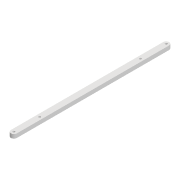
# Autodesk Inventor part: Part_5
Saved by Autodesk Inventor 2022 (Build 260153000, 153)
## iProperties
Created: 2022-04-22
Part Number: Part_5
Material: Generic
Document SubType Name: Modeling
Designer: dell
Density: 1 g/cm^3
Appearance: Default
Mass: 3.67778 g
Surface Area: 33.0626 cm^2
Volume: 3.67778 cm^3
Author: dell
Autodesk Inventor part; units mm, degrees
ref_plane "YZ Plane" through (0, 0, 0) normal (1, 0, 0) x (0, 1, 0)
ref_plane "XZ Plane" through (0, 0, 0) normal (0, 1, 0) x (-1, 0, 0)
ref_plane "XY Plane" through (0, 0, 0) normal (0, 0, 1) x (1, 0, 0)
sketch "Sketch1" plane through (0, 0, 0) normal (0, 1, 0) x (-1, 0, 0)
  line L0 (0, 0) -> (0, -153.89) construction
  line L1 (3, 0) -> (3, -153.89)
  line L2 (-3, -153.89) -> (-3, 0)
  arc A0 (3, 0) -> (-3, 0) centre (0, 0) ccw
  arc A1 (-3, -153.89) -> (3, -153.89) centre (0, -153.89) ccw
  circle A2 centre (0, 0) radius 1.1
  circle A3 centre (0, -153.89) radius 1.1
  circle A4 centre (0, -25.907) radius 1.1
  circle A5 centre (0, -127.773) radius 1.1
  point P0 (0, -76.945)
  dimension "d0" = 2.2
  dimension "d1" = 2.2
  dimension "d2" = 6
  dimension "d3" = 153.89
  dimension "d10" = 2.2
  dimension "d11" = 25.907
  dimension "d12" = 2.2
  dimension "d13" = 127.773
  constraints: 8 end point, 6 centre point, 4 point on circle, 4 tangent, 2 coincident, 2 point on line, 1 midpoint, 1 parallel, 1 vertical
  measures "d0" diameter of A2
  measures "d1" diameter of A3
  measures "d2" distance between parallel lines of L2 L1
  measures "d3" distance of L0.end L0.start
  measures "d10" diameter of A4
  measures "d11" distance of L0.start A4.centre
  measures "d12" diameter of A5
  measures "d13" distance of L0.start A5.centre
extrude "Extrusion1" add sketch "Sketch1" along normal blind 4
body "Solid1"
